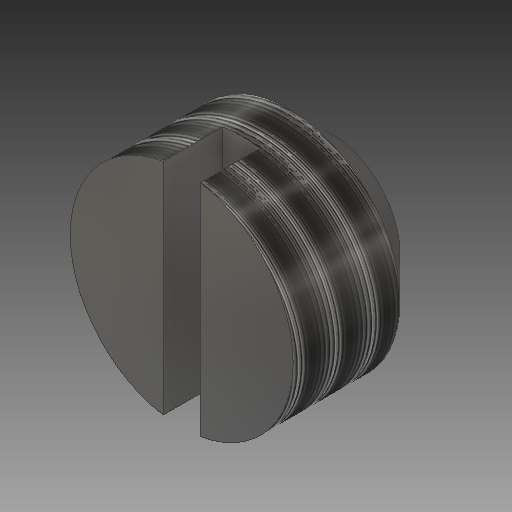
# Autodesk Inventor part: ネジ止めm3,02
Saved by Autodesk Inventor 2020 (Build 240168000, 168)
## iProperties
Created: 2018-12-29
Part Number: ネジ止めm3,02
Material: 鋼、高強度、低合金
Document SubType Name: Modeling
Designer: 雪村
Density: 7.85 g/cm^3
Appearance: 鋼 - つや出し
Mass: 0.091359 g
Surface Area: 0.333986 cm^2
Volume: 0.0116381 cm^3
Author: 雪村
Autodesk Inventor part; units mm, degrees
ref_plane "YZ Plane" through (0, 0, 0) normal (1, 0, 0) x (0, 1, 0)
ref_plane "XZ Plane" through (0, 0, 0) normal (0, 1, 0) x (-1, 0, 0)
ref_plane "XY Plane" through (0, 0, 0) normal (0, 0, 1) x (1, 0, 0)
sketch "スケッチ1" plane through (0, 0, 0) normal (0, 0, 1) x (1, 0, 0)
  circle A0 centre (0, 0) radius 1.5
  dimension "d0" = 3
  constraints: 1 centre point, 1 coincident
  measures "d0" diameter of A0
extrude "押し出し1" add sketch "スケッチ1" along normal blind 2
chamfer "面取り1" distance 0.5625 angle 45 1 edges at (-1.5, 0, 0)
thread "ねじ1" size "M3x0.5" class "6g" standard "ANSI Metric M Profile" full length
sketch "スケッチ2" plane through (0, 0, 2) normal (0, 0, 1) x (1, 0, 0)
  circle A0 centre (0, 0) radius 1.5 projected
  line L0 (-0.25, 1.479) -> (-0.25, -1.479)
  line L1 (0.25, -1.479) -> (0.25, 1.479)
  dimension "d8" = 0.25
  dimension "d9" = 0.25
  constraints: 4 end point, 4 point on circle, 2 vertical
  measures "d8" distance from line of point (0, 0) L0
  measures "d9" distance from line of L1 point (0, 0)
extrude "押し出し2" cut sketch "スケッチ2" against normal blind 0.8 contours L1 A0 L0
equation "\"d9\" = d8"
